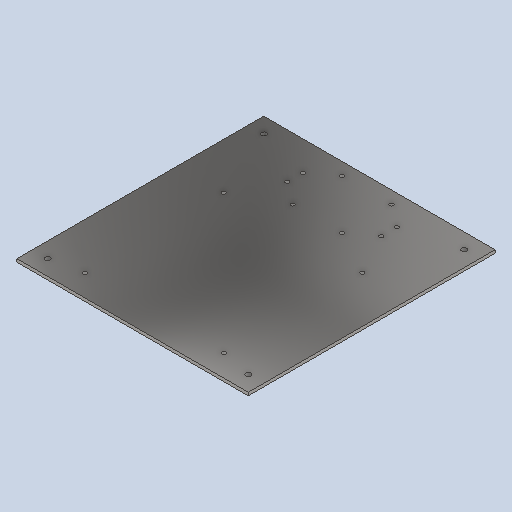
# Autodesk Inventor part: Base
Saved by Autodesk Inventor 2023 (Build 270158000, 158)
## iProperties
Created: 2023-03-17
Part Number: Base
Material: Steel
Document SubType Name: Sheet Metal
Designer: Mateus
Mass: 3532.5 g
Surface Area: 1860 cm^2
Volume: 450 cm^3
Density: 7.85 g/cm^3
Sheet Metal Rule: Default_mm
Appearance: Aço - Polido
Author: Mateus
Autodesk Inventor part; units mm, degrees
ref_plane "YZ Plane" through (0, 0, 0) normal (1, 0, 0) x (0, 1, 0)
ref_plane "XZ Plane" through (0, 0, 0) normal (0, 1, 0) x (-1, 0, 0)
ref_plane "XY Plane" through (0, 0, 0) normal (0, 0, 1) x (1, 0, 0)
sketch "Esboço1" plane through (0, 0, 0) normal (0, 1, 0) x (-1, 0, 0)
  line L0 (0, 0) -> (300, 0)
  line L1 (300, 0) -> (300, -320)
  line L2 (300, -320) -> (0, -320)
  line L3 (0, -320) -> (0, 0)
  dimension "d0" = 300
  dimension "d1" = 320
  constraints: 8 end point, 2 parallel, 1 horizontal, 1 perpendicular
  measures "d0" distance of L1.end L2.end
  measures "d1" distance of L0.end L1.end
extrude "Extrusão1" add sketch "Esboço1" along normal blind 4
sketch "Sketch4" plane through (0, 4, 0) normal (0, 1, 0) x (1, 0, 0)
  line L0 (-300, 320) -> (-300, 0) projected
  line L1 (-300, 0) -> (0, 0) projected
  line L2 (0, 320) -> (-300, 320) projected
  line L3 (0, 0) -> (0, 320) projected
  point P0 (-182, 239.6)
  point P1 (-182, 303.6)
  point P2 (-118, 239.6)
  point P3 (-118, 303.6)
  point P4 (-211, 281.6)
  point P5 (-89, 281.6)
  point P6 (-211, 261.6)
  point P7 (-89, 261.6)
  point P8 (-240, 28.1)
  point P9 (-240, 208.1)
  point P10 (-60, 28.1)
  point P11 (-60, 208.1)
  dimension "d25" = 64
  dimension "d28" = 64
  dimension "d32" = 300
  dimension "d33" = 320
  dimension "d41" = 16.4
  dimension "d42" = 118
  dimension "d45" = 122
  dimension "d48" = 20
  dimension "d51" = 38.4
  dimension "d52" = 89
  dimension "d55" = 180
  dimension "d58" = 180
  dimension "d61" = 60
  dimension "d62" = 28.1
  constraints: 3 horizontal, 3 vertical, 9 other
  measures "d25" distance of point (-182, 239.6) point (-182, 303.6)
  measures "d28" distance of point (-182, 239.6) point (-118, 239.6)
  measures "d32" distance of L0.end L1.end
  measures "d33" distance of L0.start L0.end
  measures "d41" distance from line of L2 point (-182, 303.6)
  measures "d42" distance from line of L3 point (-118, 303.6)
  measures "d45" distance of point (-211, 281.6) point (-89, 281.6)
  measures "d48" distance of point (-211, 281.6) point (-211, 261.6)
  measures "d51" distance from line of L2 point (-211, 281.6)
  measures "d52" distance from line of L0 point (-211, 261.6)
  measures "d55" distance of point (-240, 28.1) point (-240, 208.1)
  measures "d58" distance of point (-240, 28.1) point (-60, 28.1)
  measures "d61" distance from line of L0 point (-240, 28.1)
  measures "d62" distance from line of L1 point (-240, 28.1)
hole "Hole1" at (-182, 4, -239.6) at (-182, 4, -303.6) at (-118, 4, -239.6) at (-118, 4, -303.6) at (-211, 4, -261.6) at (-211, 4, -281.6) at (-89, 4, -281.6) at (-89, 4, -261.6) at (-240, 4, -28.1) at (-240, 4, -208.1) at (-60, 4, -208.1) at (-60, 4, -28.1) direction (0, -1, 0) diameter 5 end through all
sketch "Sketch5" plane through (0, 4, 0) normal (0, 1, 0) x (1, 0, 0)
  line L0 (-300, 320) -> (-300, 0) projected
  line L1 (-300, 0) -> (0, 0) projected
  point P0 (-280, 20)
  point P1 (-280, 300)
  point P2 (-20, 20)
  point P3 (-20, 300)
  dimension "d65" = 280
  dimension "d68" = 260
  dimension "d71" = 320
  dimension "d72" = 300
  dimension "d73" = 20
  dimension "d74" = 20
  constraints: 1 horizontal, 1 vertical, 3 other
  measures "d65" distance of point (-280, 20) point (-280, 300)
  measures "d68" distance of point (-280, 20) point (-20, 20)
  measures "d71" distance of L0.start L0.end
  measures "d72" distance of L0.end L1.end
  measures "d73" distance from line of L1 point (-280, 20)
  measures "d74" distance from line of L0 point (-280, 20)
hole "Hole2" at (-280, 4, -20) at (-280, 4, -300) at (-20, 4, -20) at (-20, 4, -300) direction (0, -1, 0) diameter 6.647 end through all thread size "M8x1.25" class "6H" standard "ISO Metric profile"
equation "\"d42\" = -0.5 * d28 + 0.5 * d32"
equation "\"d52\" = 0.5 * d32 - 0.5 * d45"
equation "\"d61\" = 0.5 * d32 - 0.5 * d58"
equation "\"d39\" = Espessura"
equation "\"d73\" = 0.5 * d71 - 0.5 * d65"
equation "\"d74\" = 0.5 * d72 - 0.5 * d68"
equation "\"Raio_vergadura\" = Espessura"
equation "\"Largura_alívio_de_vergadura\" = Espessura"
equation "\"Profundidade_alívio_de_vergadura\" = 0.5 * Espessura"
equation "\"Tamanho_alívio_de_dobra\" = 4 * Espessura"
equation "\"Remanescente_mínimo\" = 2 * Espessura"
equation "\"Raiodetransição\" = Raio_vergadura"
equation "\"Tamanho_de_raio_de_Jacobi\" = Raio_vergadura"
equation "\"TamanhoFolga\" = Espessura"
equation "\"Espessura\" = 0.5"
